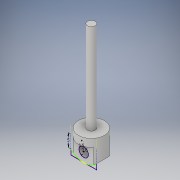
# Autodesk Inventor part: 避震
Saved by Autodesk Inventor 2019 (Build 230136000, 136)
## iProperties
Created: 2020-03-20
Part Number: 避震
Material: 一般
Document SubType Name: Modeling
Designer: 黃柏維
Density: 1 g/cm^3
Appearance: 預設
Author: 黃柏維
Autodesk Inventor part; units mm, degrees
ref_plane "YZ Plane" through (0, 0, 0) normal (1, 0, 0) x (0, 1, 0)
ref_plane "XZ Plane" through (0, 0, 0) normal (0, 1, 0) x (-1, 0, 0)
ref_plane "Work Plane1" through (-2.5, 3, 0) normal (0, 1, 0) x (1, 0, 0)
sketch "草圖8" plane through (-2.5, 3, 0) normal (0, 1, 0) x (1, 0, 0)
  circle A0 centre (2.5, -1.5) radius 5
  point P0 (2.5, 0)
  point P1 (2.5, 0)
  dimension "d26" = 10
  constraints: 4 coincident, 1 centre point
  measures "d26" diameter of A0
extrude "擠出6" add sketch "草圖8" along normal blind 3
sketch "草圖9" plane through (0, 6, 1.5) normal (0, 1, 0) x (1, 0, 0)
  circle A0 centre (0, 0) radius 1.5
  point P0 (0, 1.5)
  dimension "d29" = 3
  constraints: 1 centre point
  measures "d29" diameter of A0
extrude "擠出7" add sketch "草圖9" along normal blind 35
sketch "Sketch10" plane through (0, 3, 1.5) normal (0, -1, 0) x (1, 0, 0)
  line L0 (0, 0) -> (0, 3) construction
  circle A0 centre (0, 0) radius 5 projected
  line L1 (0, 3) -> (-4, 3)
  line L2 (0, 3) -> (4, 3)
  line L3 (0, 0) -> (0, -3) construction
  line L4 (0, -3) -> (-4, -3)
  line L5 (0, -3) -> (4, -3)
  point P0 (0, -1.5)
  dimension "d34" = 3
  dimension "d35" = 3
  constraints: 12 end point, 4 point on circle, 2 horizontal, 2 vertical, 1 perpendicular, 1 point on line
  measures "d34" distance of L0.start L0.end
  measures "d35" distance of L3.start L3.end
extrude "Extrusion8" add sketch "Sketch10" along normal blind 7 contours A0 L5 L4 L1 L2
sketch "Sketch11" plane through (-4, 3, 4.5) normal (0, 0, 1) x (1, 0, 0)
  line L0 (0, 0) -> (8, 0) construction
  line L1 (4, 0) -> (4, -3.5) construction
  circle A0 centre (4, -3.5) radius 1.8
  line L2 (-1, -7) -> (-1, 3) construction
  line L3 (-1, 0) -> (-1, -5) construction
  line L4 (9, -7) -> (9, 3) construction
  line L5 (9, 0) -> (9, -5) construction
  arc A1 (-1, -5) -> (9, -5) centre (4, 0) ccw
  line L6 (-1, -7) -> (0, -7) projected
  line L7 (-1, -5) -> (-1, -7)
  line L8 (8, -7) -> (9, -7) projected
  line L9 (9, -7) -> (9, -5)
  line L10 (-1, -7) -> (3, -7)
  line L11 (8, -7) -> (0, -7) projected
  line L12 (9, -7) -> (5, -7)
  point P0 (4, -3)
  dimension "d38" = 3.5
  dimension "d39" = 3.6
  dimension "d40" = 5
  constraints: 14 end point, 5 point on line, 4 point on circle, 2 centre point, 2 coincident, 2 collinear, 2 vertical, 1 midpoint
  measures "d38" distance of L1.start L1.end
  measures "d39" diameter of A0
  measures "d40" distance of L3.start L3.end
extrude "Extrusion9" cut sketch "Sketch11" against normal through all contours A0
extrude "Extrusion10" cut sketch "Sketch11" against normal blind 7 contours A1 L9 L8 L11 | A1 L10 L6 L7
equation "\"d41\" = d38"
